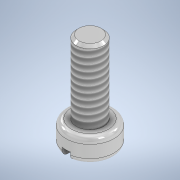
# Autodesk Inventor part: connector_screw
Saved by Autodesk Inventor 2021 (Build 250183000, 183)
## iProperties
Created: 2022-03-25
Part Number: connector_screw
Material: Aluminum 6061-AHC
Document SubType Name: Modeling
Designer: ermoz
Density: 2.7 g/cm^3
Appearance: Aluminum - Dark
Author: ermoz
Autodesk Inventor part; units mm, degrees
ref_plane "YZ Plane" through (0, 0, 0) normal (1, 0, 0) x (0, 1, 0)
ref_plane "XZ Plane" through (0, 0, 0) normal (0, 1, 0) x (-1, 0, 0)
ref_plane "XY Plane" through (0, 0, 0) normal (0, 0, 1) x (1, 0, 0)
sketch "Sketch1" plane through (0, 0, 0) normal (0, 1, 0) x (-1, 0, 0)
  circle A0 centre (0, 0) radius 1.75
  dimension "d0" = 3.5
  constraints: 1 centre point, 1 coincident
  measures "d0" diameter of A0
extrude "Extrusion1" add sketch "Sketch1" along normal blind 1.7
sketch "Sketch2" plane through (0, 1.7, 0) normal (0, 1, 0) x (1, 0, 0)
  circle A0 centre (0, 0) radius 1
  dimension "d3" = 2
  constraints: 1 centre point, 1 coincident
  measures "d3" diameter of A0
extrude "Extrusion2" add sketch "Sketch2" along normal blind 5.3
thread "Thread1" size "M2.5x0.45" class "6g" standard "ANSI Metric M Profile" full length
fillet "Fillet1" radius 0.4 2 edges at (1.75, 1.7, 0) (1.75, 0, 0)
sketch "Sketch3" plane through (0, 0, 0) normal (0, -1, 0) x (1, 0, 0)
  line L0 (-0.3, -1.75) -> (0.3, -1.75)
  line L1 (0.3, -1.75) -> (0.3, 1.75)
  line L2 (0.3, 1.75) -> (-0.3, 1.75)
  line L3 (-0.3, 1.75) -> (-0.3, -1.75)
  line L4 (-0.3, -1.75) -> (0.3, 1.75) construction
  line L5 (0.3, -1.75) -> (-0.3, 1.75) construction
  circle A0 centre (0, 0) radius 1.75 projected
  point P0 (0.3, -1.7241)
  point P1 (0.3, 1.7241)
  point P2 (-0.3, 1.7241)
  point P3 (-0.3, -1.7241)
  dimension "d9" = 0.6
  constraints: 12 end point, 2 midpoint, 2 parallel, 1 horizontal, 1 perpendicular, 1 tangent
  measures "d9" distance of L2.end L1.end
extrude "Extrusion3" cut sketch "Sketch3" against normal blind 0.6 contours A0 L3 L1
chamfer "Chamfer1" distance 0.2 angle 45 1 edges at (-1, 7, 0)
body "Solid1"
